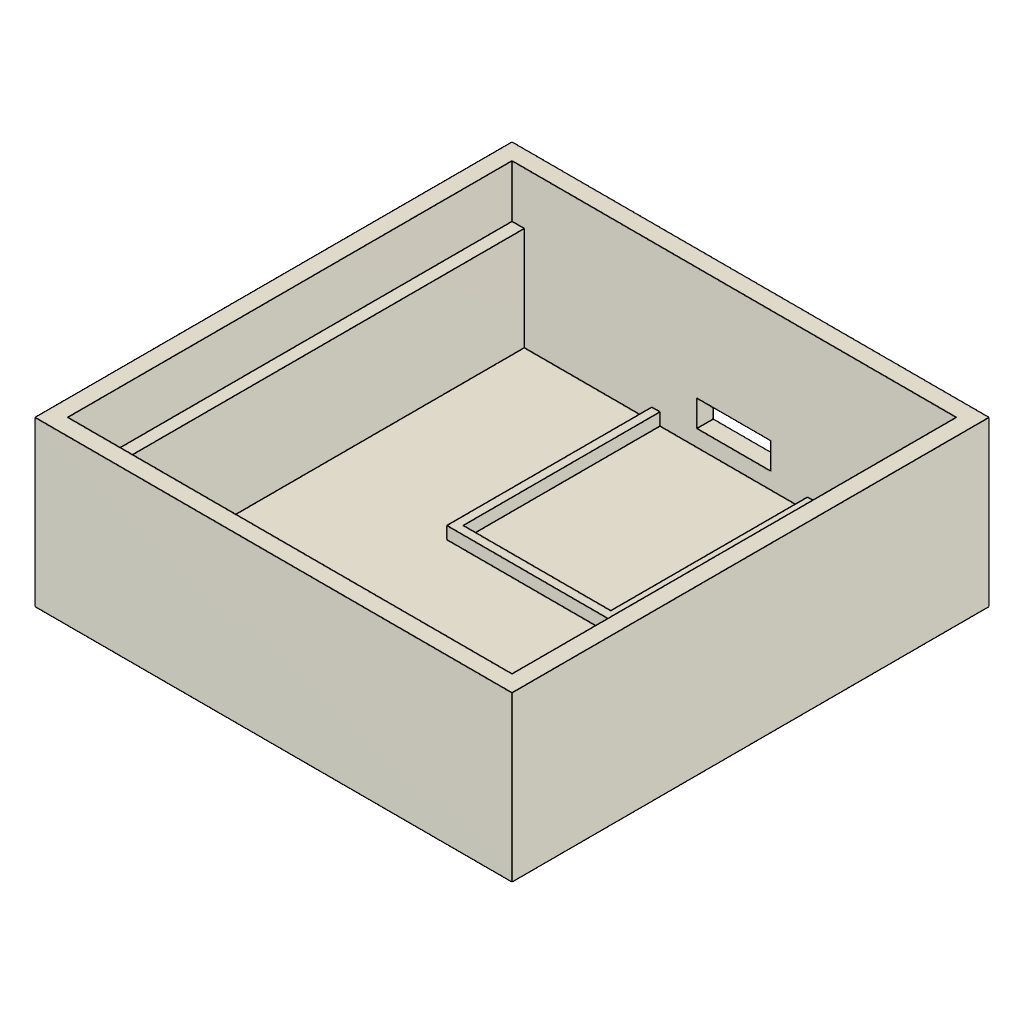
assembly (Autodesk Fusion 360 archive; units mm, degrees)
design "case"
part number: 2026-10-06-01-14-02-929
Autodesk Fusion 360 part; units mm, degrees
sketch "Sketch1" plane through (0, 0, 0) normal (0, 1, 0) x (1, 0, 0)
  line L0 (0, 0) -> (54.2, 0)
  line L1 (54.2, 0) -> (54.2, 54.2)
  line L2 (54.2, 54.2) -> (0, 54.2)
  line L3 (0, 54.2) -> (0, 0)
  line L4 (-2, -2) -> (56.2, -2)
  line L5 (56.2, -2) -> (56.2, 56.2)
  line L6 (56.2, 56.2) -> (-2, 56.2)
  line L7 (-2, 56.2) -> (-2, -2)
  line L8 (1.5, 54.2) -> (1.5, 0)
  line L9 (52.7, 54.2) -> (52.7, 0)
  dimension "d1" = 54.2
  dimension "d2" = 54.2
  dimension "d3" = 2
  dimension "d15" = 1.5
  dimension "d16" = 1.5
  constraint horizontal L0
  constraint vertical L1
  constraint horizontal L2
  constraint vertical L3
  constraint coincident L0.start L3.end
  constraint coincident L2 L8.start
  constraint coincident L0 L8.end
  constraint perpendicular L0 L8
  constraint coincident L2 L9.start
  constraint coincident L0 L9.end
  constraint perpendicular L0 L9
  measures "d1" distance of L0.start L2.end
  measures "d2" distance of L1.end L2.end
  measures "d15" distance of L3 L8
  measures "d16" distance of L1 L9
extrude "Extrude3" add sketch "Sketch1" along normal blind 13.6 contours L0 L2 L3 L8 | L0 L1 L2 L9 makes body 1 at (52.7, 4.5333, -36.1333) makes body 2 at (0, 4.5333, -36.1333)
extrude "Extrude1" add sketch "Sketch1" along normal blind 1 contours L0 L2 L3 L8 | L0 L2 L8 L9 | L0 L1 L2 L9 bodies 1 2
extrude "Extrude2" add sketch "Sketch1" along normal blind 20 bodies 1
sketch "Sketch2" plane through (0, 1, 0) normal (0, 1, 0) x (-1, 0, 0)
  line L0 (-52.7, 0) -> (-52.7, -54.2)
  line L1 (-52.7, -54.2) -> (-1.5, -54.2)
  line L2 (-1.5, -54.2) -> (-1.5, 0)
  line L3 (-1.5, 0) -> (-52.7, 0)
  line L4 (-1.5, -54.2) -> (-52.7, -54.2) construction
  line L5 (-18.05, -54.2) -> (-36.05, -54.2)
  line L6 (-36.05, -54.2) -> (-36.05, -30.2)
  line L7 (-36.05, -30.2) -> (-18.05, -30.2)
  line L8 (-18.05, -30.2) -> (-18.05, -54.2)
  line L9 (-17.05, -54.2) -> (-17.05, -29.2)
  line L10 (-17.05, -29.2) -> (-37.05, -29.2)
  line L11 (-37.05, -29.2) -> (-37.05, -54.2)
  dimension "d18" = 24
  dimension "d19" = 18
  dimension "d20" = 16.55
  dimension "d21" = 16.65
  dimension "d22" = 1
  dimension "d23" = 1
  dimension "d24" = 1
  constraint coincident L1.end L2.start
  constraint coincident L0.end L1.start
  constraint horizontal L5
  constraint vertical L6
  constraint horizontal L7
  constraint vertical L8
  constraint coincident L4 L5.start
  constraint coincident L4 L9.start
  constraint perpendicular L4 L9
  constraint perpendicular L9 L10
  constraint coincident L4 L11.end
  constraint perpendicular L4 L11
  measures "d18" distance of L5 L7
  measures "d19" distance of L6 L8
  measures "d20" distance of L2 L8
  measures "d21" distance of L0 L6
  measures "d22" distance of L8 L9
  measures "d23" distance of L7 L10
  measures "d24" distance of L6 L11
extrude "Extrude4" add sketch "Sketch2" along normal blind 1.5 contours L1 L6 L7 L8 L9 L10 L11 bodies 1
sketch "Sketch3" plane through (0, 0, -56.2) normal (0, 0, -1) x (-1, 0, 0)
  line L0 (-56.2, 0) -> (2, 0)
  line L1 (2, 0) -> (2, 20)
  line L2 (2, 20) -> (-56.2, 20)
  line L3 (-56.2, 20) -> (-56.2, 0)
  line L4 (-31.55, 6.2) -> (-22.55, 6.2)
  line L5 (-22.55, 6.2) -> (-22.55, 3)
  line L6 (-22.55, 3) -> (-31.55, 3)
  line L7 (-31.55, 3) -> (-31.55, 6.2)
  dimension "d27" = 9
  dimension "d28" = 3.2
  dimension "d29" = 24.55
  dimension "d30" = 24.65
  dimension "d31" = 3
  constraint horizontal L4
  constraint vertical L5
  constraint horizontal L6
  constraint vertical L7
  measures "d27" distance of L4.start L4.end
  measures "d28" distance of L4.start L6.end
  measures "d29" distance of L1 L5
  measures "d30" distance of L3 L7
  measures "d31" distance of L0 L6
extrude "Extrude5" cut sketch "Sketch3" against normal up to surface (2 mm away) contours L4 L5 L6 L7 bodies 1
equation "d9 = 20 mm - 6.4 mm"
equation "d23 = d22"
equation "d24 = d23"

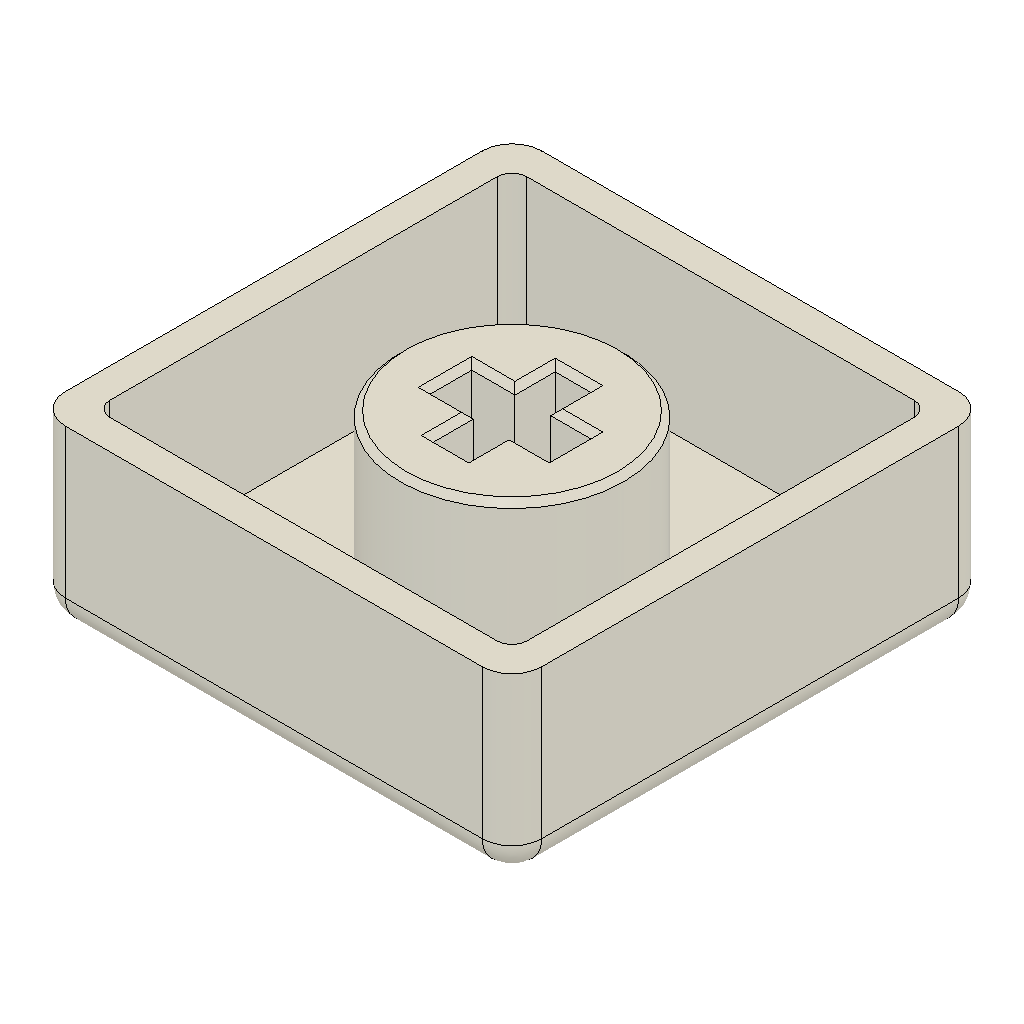
design "keycaps"
part number: 2026-10-06-00-52-50-519
Autodesk Fusion 360 part; units mm, degrees
sketch "Sketch1" plane through (0, 0, 0) normal (0, 1, 0) x (1, 0, 0)
  line L0 (0, 0) -> (16, 0)
  line L1 (16, 0) -> (16, 16)
  line L2 (16, 16) -> (0, 16)
  line L3 (0, 16) -> (0, 0)
  dimension "d1" = 16
  dimension "d2" = 16
  constraint horizontal L0
  constraint vertical L1
  constraint horizontal L2
  constraint vertical L3
  constraint coincident L0.start L3.end
  measures "d1" distance of L0.start L0.end
  measures "d2" distance of L0.start L2.end
extrude "Extrude1" add sketch "Sketch1" along normal blind 1
sketch "Sketch2" plane through (0, 1, 0) normal (0, 1, 0) x (-1, 0, 0)
  line L0 (0, -16) -> (0, 0)
  line L1 (0, 0) -> (-16, 0)
  line L2 (-16, 0) -> (-16, -16)
  line L3 (-16, -16) -> (0, -16)
  line L4 (-7.45, -10) -> (-8.65, -10)
  line L5 (-8.65, -10) -> (-8.65, -8.65)
  line L6 (-8.65, -8.65) -> (-10, -8.65)
  line L7 (-10, -8.65) -> (-10, -7.25)
  line L8 (-10, -7.25) -> (-8.65, -7.25)
  line L9 (-8.65, -7.25) -> (-8.65, -5.9)
  line L10 (-8.65, -5.9) -> (-7.45, -5.9)
  line L11 (-7.45, -5.9) -> (-7.45, -7.25)
  line L12 (-7.45, -7.25) -> (-6, -7.25)
  line L13 (-6, -7.25) -> (-6, -8.65)
  line L14 (-6, -8.65) -> (-7.45, -8.65)
  line L15 (-7.45, -8.65) -> (-7.45, -10)
  line L16 (-7.45, -8.65) -> (-8.65, -7.25) construction
  line L17 (-8.65, -8.65) -> (-7.45, -7.25) construction
  circle A0 centre (-8.05, -7.95) radius 3.75
  dimension "d5" = 4
  dimension "d6" = 1.45
  dimension "d7" = 1.35
  dimension "d8" = 1.4
  dimension "d9" = 1.2
  dimension "d10" = 1.35
  dimension "d11" = 6
  dimension "d12" = 5.9
  dimension "d13" = 6
  dimension "d14" = 6
  dimension "d15" = 7.5
  dimension "d27" = 16
  constraint horizontal L4
  constraint perpendicular L4 L5
  constraint perpendicular L5 L6
  constraint vertical L7
  constraint perpendicular L7 L8
  constraint perpendicular L8 L9
  constraint perpendicular L7 L10
  constraint perpendicular L10 L11
  constraint perpendicular L11 L12
  constraint perpendicular L12 L13
  constraint perpendicular L11 L14
  constraint vertical L15
  constraint collinear L11 L15
  constraint collinear L5 L9
  constraint collinear L8 L12
  constraint collinear L6 L14
  constraint midpoint L17 A0.centre
  measures "d5" distance of L7 L13
  measures "d6" distance of L13.end L14.end
  measures "d7" distance of L4.start L14.end
  measures "d8" distance of L12.end L13.end
  measures "d9" distance of L4.start L4.end
  measures "d10" distance of L10.end L11.end
  measures "d11" distance of L3 L4
  measures "d12" distance of L1 L10
  measures "d13" distance of L2 L7
  measures "d14" distance of L0 L13
  measures "d15" diameter of A0
  measures "d27" distance of L0 L2
extrude "Extrude2" add sketch "Sketch2" along normal blind 5 contours A0
sketch "Sketch3" plane through (0, 1, 0) normal (0, 1, 0) x (-1, 0, 0)
  line L0 (0, -16) -> (0, 0)
  line L1 (0, 0) -> (-16, 0)
  line L2 (-16, 0) -> (-16, -16)
  line L3 (-16, -16) -> (0, -16)
  circle A0 centre (-8.05, -7.95) radius 3.75
  line L4 (0, -16) -> (-16, -16)
  line L5 (-16, -16) -> (-16, 0)
  line L6 (-16, 0) -> (0, 0)
  line L7 (0, 0) -> (0, -16)
  line L8 (-15, -1) -> (-1, -1)
  line L9 (-1, -1) -> (-1, -15)
  line L10 (-1, -15) -> (-15, -15)
  line L11 (-15, -15) -> (-15, -1)
  dimension "d18" = 1
  constraint horizontal L4
  constraint vertical L5
  constraint horizontal L6
  constraint vertical L7
  constraint coincident L1.end L2.start
  constraint coincident L0.start L3.end
extrude "Extrude3" add sketch "Sketch3" along normal blind 5 contours L0 L1 L2 L3 L4 L5 L6 L7
chamfer "Chamfer1" distance 0.2 angle 45 12 edges at (7.45, 6, -9.325) (8.05, 6, -10) (8.65, 6, -9.325) (9.325, 6, -8.65) (10, 6, -7.95) (9.325, 6, -7.25) (8.65, 6, -6.575) (8.05, 6, -5.9) (7.45, 6, -6.575) (6.725, 6, -7.25) (6, 6, -7.95) (6.725, 6, -8.65)
chamfer "Chamfer1" distance 0.2 angle 45 1 edges at (11.5462, 6, -9.3061)
fillet "Fillet1" radius 1 4 edges at (0, 3, -16) (0, 3, 0) (16, 3, 0) (16, 3, -16) 1 faces at (5.3333, 0, -5.3333)
fillet "Fillet1" radius 0.5 4 edges at (1, 3.5, -15) (1, 3.5, -1) (15, 3.5, -1) (15, 3.5, -15)
equation "d10 = d7"

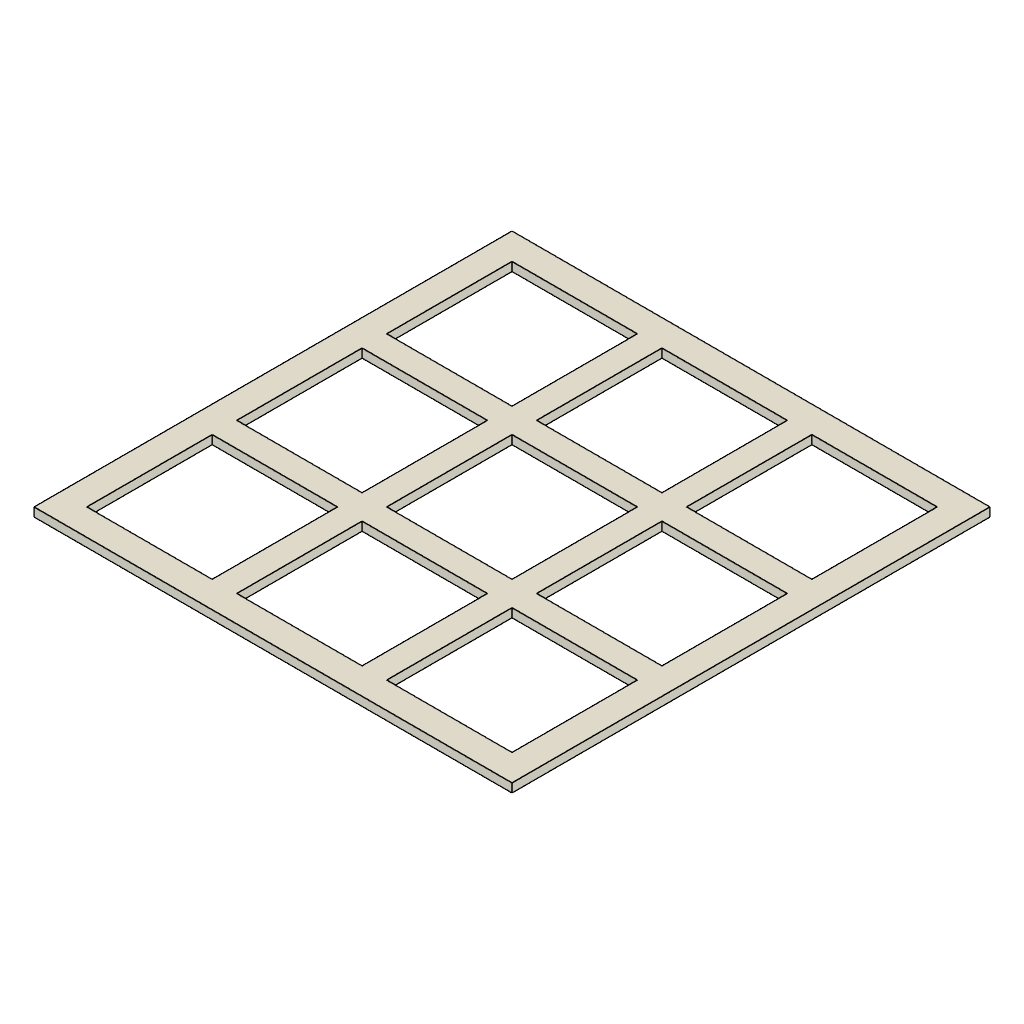
design "socket"
part number: 2026-10-06-00-32-47-322
Autodesk Fusion 360 part; units mm, degrees
sketch "Sketch1" plane through (0, 0, 0) normal (0, 1, 0) x (1, 0, 0)
  line L0 (0, 0) -> (14.2, 0)
  line L1 (14.2, 0) -> (14.2, 14.2)
  line L2 (14.2, 14.2) -> (0, 14.2)
  line L3 (0, 14.2) -> (0, 0)
  line L4 (17, 14.2) -> (17, 0)
  line L5 (31.2, 0) -> (31.2, 14.2)
  line L6 (17, 0) -> (31.2, 0)
  line L7 (31.2, 14.2) -> (17, 14.2)
  line L8 (34, 14.2) -> (34, 0)
  line L9 (48.2, 0) -> (48.2, 14.2)
  line L10 (34, 0) -> (48.2, 0)
  line L11 (48.2, 14.2) -> (34, 14.2)
  line L12 (0, 31.2) -> (0, 17)
  line L13 (14.2, 17) -> (14.2, 31.2)
  line L14 (0, 17) -> (14.2, 17)
  line L15 (14.2, 31.2) -> (0, 31.2)
  line L16 (17, 31.2) -> (17, 17)
  line L17 (31.2, 17) -> (31.2, 31.2)
  line L18 (17, 17) -> (31.2, 17)
  line L19 (31.2, 31.2) -> (17, 31.2)
  line L20 (34, 31.2) -> (34, 17)
  line L21 (48.2, 17) -> (48.2, 31.2)
  line L22 (34, 17) -> (48.2, 17)
  line L23 (48.2, 31.2) -> (34, 31.2)
  line L24 (0, 48.2) -> (0, 34)
  line L25 (14.2, 34) -> (14.2, 48.2)
  line L26 (0, 34) -> (14.2, 34)
  line L27 (14.2, 48.2) -> (0, 48.2)
  line L28 (17, 48.2) -> (17, 34)
  line L29 (31.2, 34) -> (31.2, 48.2)
  line L30 (17, 34) -> (31.2, 34)
  line L31 (31.2, 48.2) -> (17, 48.2)
  line L32 (34, 48.2) -> (34, 34)
  line L33 (48.2, 34) -> (48.2, 48.2)
  line L34 (34, 34) -> (48.2, 34)
  line L35 (48.2, 48.2) -> (34, 48.2)
  line L36 (-3, -3) -> (51.2, -3)
  line L37 (51.2, -3) -> (51.2, 51.2)
  line L38 (51.2, 51.2) -> (-3, 51.2)
  line L39 (-3, 51.2) -> (-3, -3)
  point P0 (17, 0)
  point P1 (34, 0)
  point P2 (0, 17)
  point P3 (17, 17)
  point P4 (34, 17)
  point P5 (0, 34)
  point P6 (17, 34)
  point P7 (34, 34)
  dimension "d1" = 14.2
  dimension "d2" = 14.2
  dimension "d5" = 17
  dimension "d6" = 17
  dimension "d7" = 3
  dimension "d8" = 3
  dimension "d9" = 3
  dimension "d10" = 3
  constraint horizontal L0
  constraint vertical L1
  constraint horizontal L2
  constraint vertical L3
  constraint coincident L0.start L3.end
  constraint horizontal L36
  constraint vertical L37
  constraint horizontal L38
  constraint vertical L39
  measures "d1" distance of L1.end L2.end
  measures "d2" distance of L0.end L1.end
  measures "d7" distance of L0 L36
  measures "d8" distance of L3 L39
  measures "d9" distance of L9 L37
  measures "d10" distance of L35 L38
extrude "Extrude1" add sketch "Sketch1" along normal blind 1
